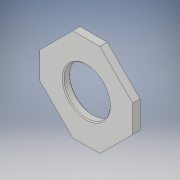
# Autodesk Inventor part: support_bois_reservoir
Saved by Autodesk Inventor 2019 (Build 230136000, 136)
## iProperties
Created: 2018-05-09
Part Number: support_bois_reservoir
Material: Générique
Document SubType Name: Modeling
Designer: Theo
Density: 1 g/cm^3
Appearance: Par défaut
Author: Theo
Autodesk Inventor part; units mm, degrees
ref_plane "YZ Plane" through (0, 0, 0) normal (1, 0, 0) x (0, 1, 0)
ref_plane "XZ Plane" through (0, 0, 0) normal (0, 1, 0) x (-1, 0, 0)
ref_plane "XY Plane" through (0, 0, 0) normal (0, 0, 1) x (1, 0, 0)
sketch "Esquisse1" plane through (0, 0, 0) normal (0, 0, 1) x (1, 0, 0)
  circle A0 centre (0, 0) radius 25
  line L0 (-50, 14.6447) -> (-14.6447, 50)
  line L1 (14.6447, 50) -> (50, 14.6447)
  line L2 (50, -14.6447) -> (14.6447, -50)
  line L3 (-14.6447, -50) -> (-50, -14.6447)
  line L4 (-70, 0) -> (70, 0) construction
  line L5 (0, -70) -> (0, 70) construction
  line L6 (50, -14.6447) -> (50, 14.6447)
  line L7 (-50, -14.6447) -> (-50, 14.6447)
  line L8 (-14.6447, 50) -> (14.6447, 50)
  line L9 (-14.6447, -50) -> (14.6447, -50)
  dimension "d0" = 50
  dimension "d9" = 100
  dimension "d11" = 45
  dimension "d12" = 50
  dimension "d13" = 100
  dimension "d14" = 50
  dimension "d15" = 50
  constraints: 16 end point, 3 equal length, 2 horizontal, 2 parallel, 2 vertical, 1 centre point, 1 coincident, 1 perpendicular
  measures "d0" diameter of A0
  measures "d9" distance between parallel lines of L6 L7
  measures "d11" angle of L1 L6
  measures "d12" horizontal distance of L1.end point (0, 0)
  measures "d13" distance between parallel lines of L9 L8
  measures "d14" distance from line of L4 L3.start
  measures "d15" distance of L2.start L2.end
extrude "Extrusion1" add sketch "Esquisse1" along normal blind 8
chamfer "Chanfrein1" distance 1 angle 45 2 edges at (-25, 0, 8) (-25, 0, 0)
equation "\"d12\" = 0.5 * d9"
equation "\"d13\" = d9"
equation "\"d14\" = 0.5 * d13"
